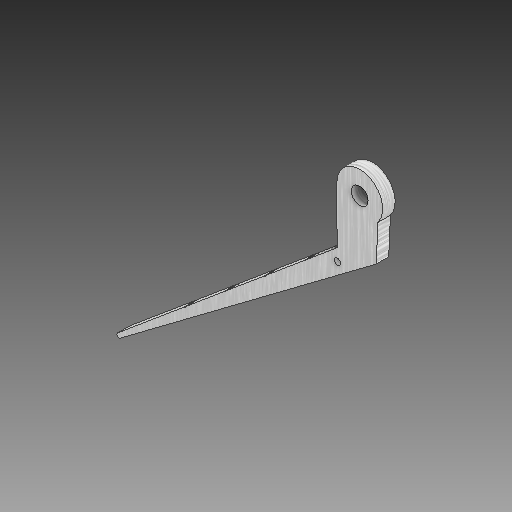
# Autodesk Inventor part: アームシールド根本1
Saved by Autodesk Inventor 2020 (Build 240168000, 168)
## iProperties
Created: 2019-09-16
Part Number: アームシールド根本1
Material: アルミニウム 7075
Document SubType Name: Modeling
Designer: 雪村
Density: 2.81 g/cm^3
Appearance: サテン - ブラシ仕上げ 重厚
Mass: 24.6363 g
Surface Area: 56.0611 cm^2
Volume: 8.76735 cm^3
Author: 雪村
Autodesk Inventor part; units mm, degrees
ref_plane "YZ Plane" through (0, 0, 0) normal (1, 0, 0) x (0, 1, 0)
ref_plane "XZ Plane" through (0, 0, 0) normal (0, 1, 0) x (-1, 0, 0)
ref_plane "XY Plane" through (0, 0, 0) normal (0, 0, 1) x (1, 0, 0)
sketch "スケッチ1" plane through (0, 0, 0) normal (0, 0, 1) x (1, 0, 0)
  circle A0 centre (-149.101, -13.3308) radius 1.5 construction
  circle A1 centre (-160.5892, -1.6149) radius 1.5 construction
  circle A2 centre (-44.4492, 64.0137) radius 1.5 construction
  circle A3 centre (-64.4423, 49.0046) radius 1.5 construction
  circle A4 centre (-60.4494, 64.5064) radius 1.5 construction
  arc A5 (-40.2316, 58.3956) -> (-44.233, 71.0354) centre (-44.4492, 64.0137) ccw construction
  line L0 (-44.233, 71.0354) -> (-60.2332, 71.5281) construction
  arc A6 (-60.2332, 71.5281) -> (-64.1725, 70.4637) centre (-60.4494, 64.5064) ccw construction
  line L1 (-64.1725, 70.4637) -> (-165.9022, 6.8864) construction
  arc A7 (-165.9022, 6.8864) -> (-166.8262, -9.4635) centre (-160.5892, -1.6149) ccw construction
  line L2 (-166.8262, -9.4635) -> (-154.0782, -19.594) construction
  arc A8 (-154.0782, -19.594) -> (-144.2981, -19.7286) centre (-149.101, -13.3308) ccw construction
  line L3 (-144.2981, -19.7286) -> (-40.2316, 58.3956) construction
  circle A9 centre (-82.1645, 51.5544) radius 1.5 construction
  circle A10 centre (-141.748, 14.817) radius 1.5 construction
  circle A11 centre (-89.4637, 29.5642) radius 1.5 construction
  circle A12 centre (-117.4541, 8.5514) radius 1.5 construction
  circle A13 centre (-111.8449, 33.0052) radius 1.5 construction
  line L4 (-152.7009, -26.0367) -> (-305.9655, -141.0946)
  circle A14 centre (-149.101, -13.3308) radius 1.5 construction
  circle A15 centre (-149.101, -13.3308) radius 3 construction
  circle A16 centre (-149.101, -13.3308) radius 3 construction
  circle A17 centre (-160.5892, -1.6149) radius 9.025 construction
  circle A18 centre (-160.5892, -1.6149) radius 4.025
  line L5 (-152.7009, -26.0367) -> (-151.5741, -2.0382)
  line L6 (-64.1725, 70.4637) -> (-165.9022, 6.8864) construction
  line L7 (-144.2981, -19.7286) -> (-40.2316, 58.3956) construction
  line L8 (-305.9655, -141.0946) -> (-171.4423, -28.6314)
  line L9 (-160.5892, -1.6149) -> (-146.0204, -21.0215) construction
  line L10 (-146.0204, -21.0215) -> (-305.9655, -141.0946) construction
  circle A19 centre (-276.0256, -117.3678) radius 1
  circle A20 centre (-160.5892, -1.6149) radius 11
  line L11 (-171.4423, -28.6314) -> (-171.589, -1.6748)
  point P0 (0, 0)
  point P1 (0, 0)
  point P2 (-276.667, -116.6006)
  point P3 (-275.4252, -118.1676)
  point P4 (-151.8691, -8.3201)
  dimension "d6" = 22
  dimension "d0" = 6
  dimension "d1" = 8.05
  dimension "d2" = 5
  dimension "d3" = 3
  dimension "d4" = 200
  dimension "d5" = 2
  dimension "d7" = 3
  dimension "d8" = 6
  constraints: 24 end point, 19 centre point, 8 point on circle, 4 tangent, 3 coincident, 2 collinear, 2 concentric, 1 perpendicular, 42 other
  measures "d0" diameter of A15
  measures "d1" diameter of A18
  measures "d3" angle of L4 L8
  measures "d4" distance of L9.end L4.end
  measures "d5" diameter of A19
  measures "d7" angle of L5 L11
  measures "d8" diameter of A16
extrude "押し出し1" add sketch "スケッチ1" along normal blind 6 contours L4 A19 L8 L11 A20 L5 | A19 | A20
sketch "スケッチ2" plane through (0, 0, 6) normal (0, 0, 1) x (1, 0, 0)
  line L0 (-171.589, -1.6748) -> (-171.4423, -28.6314) projected
  line L1 (-171.4423, -28.6314) -> (-276.667, -116.6006) projected
  arc A0 (-276.667, -116.6006) -> (-275.4252, -118.1676) centre (-276.0256, -117.3678) ccw projected
  line L2 (-275.4252, -118.1676) -> (-152.7009, -26.0367) projected
  line L3 (-152.7009, -26.0367) -> (-151.8691, -8.3201) projected
  arc A1 (-151.8691, -8.3201) -> (-171.589, -1.6748) centre (-160.5892, -1.6149) ccw projected
  circle A2 centre (-160.5892, -1.6149) radius 4.025 projected
  circle A3 centre (-171.2358, -34.3242) radius 1.5
  circle A4 centre (-171.2358, -34.3242) radius 3
  circle A5 centre (-171.2358, -34.3242) radius 4.5
  point P0 (0, 0)
  dimension "d11" = 3
  dimension "d12" = 6
  dimension "d13" = 9
  constraints: 3 centre point, 2 coincident, 2 tangent
  measures "d11" diameter of A3
  measures "d12" diameter of A4
  measures "d13" diameter of A5
extrude "押し出し2" cut sketch "スケッチ2" against normal through all contours A3
sketch "スケッチ3" plane through (0, 0, 6) normal (0, 0, 1) x (1, 0, 0)
  line L0 (-171.4423, -28.6314) -> (-276.667, -116.6006) projected
  circle A0 centre (-244.7975, -88.9797) radius 1.05
  circle A1 centre (-225.6172, -72.9448) radius 1.05
  circle A2 centre (-206.437, -56.9099) radius 1.05
  circle A3 centre (-187.2568, -40.8749) radius 1.05
  point P0 (0, 0)
  dimension "d16" = 2.1
  dimension "d17" = 2.1
  dimension "d18" = 2.1
  dimension "d19" = 2.1
  dimension "d20" = 0.75
  dimension "d21" = 0.75
  dimension "d22" = 0.75
  dimension "d23" = 0.75
  dimension "d24" = 20
  dimension "d25" = 25
  dimension "d26" = 25
  dimension "d27" = 25
  constraints: 4 centre point
  measures "d16" diameter of A0
  measures "d17" diameter of A1
  measures "d18" diameter of A2
  measures "d19" diameter of A3
  measures "d20" distance from line of L0 A3.centre
  measures "d21" distance from line of L0 A2.centre
  measures "d22" distance from line of L0 A0.centre
  measures "d23" distance from line of L0 A1.centre
  measures "d24" distance of A3.centre L0.start
  measures "d25" distance of A2.centre A3.centre
  measures "d26" distance of A1.centre A2.centre
  measures "d27" distance of A1.centre A0.centre
extrude "押し出し3" cut sketch "スケッチ3" against normal through all
sketch "スケッチ4" plane through (-205.3922, -57.0139, 6) normal (-0.6413971, 0.7672091, 0) x (0.7672091, 0.6413971, 0)
  line L0 (-25, 6) -> (-25, 0) projected
  line L1 (-1.4697, 0) -> (-25, 0) projected
  line L2 (-1.4697, 0) -> (-1.4697, 6) projected
  line L3 (-1.4697, 6) -> (-25, 6) projected
  line L4 (-26.4697, 0) -> (-26.4697, 6) projected
  line L5 (-26.4697, 6) -> (-50, 6) projected
  line L6 (-50, 6) -> (-50, 0) projected
  line L7 (-26.4697, 0) -> (-50, 0) projected
  line L8 (-51.4697, 0) -> (-51.4697, 6) projected
  line L9 (-51.4697, 6) -> (-92.9014, 6) projected
  line L10 (-92.9014, 6) -> (-92.9014, 0) projected
  line L11 (-51.4697, 0) -> (-92.9014, 0) projected
  line L12 (0, 6) -> (0, 0) projected
  line L13 (23.5303, 0) -> (0, 0) projected
  line L14 (23.5303, 0) -> (23.5303, 6) projected
  line L15 (23.5303, 6) -> (0, 6) projected
  line L16 (25, 6) -> (25, 0) projected
  line L17 (44.2511, 0) -> (25, 0) projected
  line L18 (44.2511, 6) -> (44.2511, 0) projected
  line L19 (44.2511, 6) -> (25, 6) projected
  circle A0 centre (-50.7348, 3) radius 1.25
  circle A1 centre (-25.7348, 3) radius 1.25
  circle A2 centre (-0.7348, 3) radius 1.25
  circle A3 centre (24.2652, 3) radius 1.25
  line L20 (23.5303, 6) -> (25, 6) projected
  line L21 (-1.4697, 6) -> (0, 6) projected
  line L22 (-26.4697, 6) -> (-25, 6) projected
  line L23 (-51.4697, 6) -> (-50, 6) projected
  point P0 (194.1473, 6)
  point P1 (-51.4697, 3)
  point P2 (-26.4697, 3)
  point P3 (-50.7348, 6)
  point P4 (-25.7348, 6)
  point P5 (-0.7348, 6)
  point P6 (24.2652, 6)
  point P7 (23.5303, 3)
  point P8 (-1.4697, 3)
  dimension "d30" = 2.5
  dimension "d31" = 2.5
  dimension "d32" = 2.5
  dimension "d33" = 2.5
  constraints: 8 midpoint, 4 centre point, 4 horizontal alignment, 4 vertical alignment
  measures "d30" diameter of A0
  measures "d31" diameter of A1
  measures "d32" diameter of A2
  measures "d33" diameter of A3
extrude "押し出し4" cut sketch "スケッチ4" against normal through all contours A1 L0 | L0 A1 L4 | L4 A1 | A2 L12 L2 | L2 A2 | A2 L12 | A0 L6 | L6 A0 L8 | A3 L16 L14 | L14 A3 | L8 A0 | A3 L16
sketch "スケッチ5" plane through (0, 0, 6) normal (0, 0, 1) x (1, 0, 0)
  arc A0 (-225.7, -73.9915) -> (-224.5724, -73.0489) centre (-225.6172, -72.9448) ccw projected
  line L0 (-225.7, -73.9915) -> (-243.7526, -89.0838) projected
  arc A1 (-244.8802, -90.0264) -> (-243.7526, -89.0838) centre (-244.7975, -88.9797) ccw projected
  line L1 (-244.8802, -90.0264) -> (-276.667, -116.6006) projected
  arc A2 (-276.667, -116.6006) -> (-275.4252, -118.1676) centre (-276.0256, -117.3678) ccw projected
  line L2 (-275.4252, -118.1676) -> (-152.7009, -26.0367) projected
  line L3 (-152.7009, -26.0367) -> (-151.8691, -8.3201) projected
  arc A3 (-151.8691, -8.3201) -> (-171.589, -1.6748) centre (-160.5892, -1.6149) ccw projected
  line L4 (-171.589, -1.6748) -> (-171.4423, -28.6314) projected
  line L5 (-171.4423, -28.6314) -> (-186.2119, -40.979) projected
  arc A4 (-187.3395, -41.9217) -> (-186.2119, -40.979) centre (-187.2568, -40.8749) ccw projected
  line L6 (-187.3395, -41.9217) -> (-205.3922, -57.0139) projected
  arc A5 (-206.5197, -57.9566) -> (-205.3922, -57.0139) centre (-206.437, -56.9099) ccw projected
  line L7 (-206.5197, -57.9566) -> (-224.5724, -73.0489) projected
  circle A6 centre (-171.2358, -34.3242) radius 1.5 projected
  circle A7 centre (-160.5892, -1.6149) radius 4.025 projected
  point P0 (0, 0)
equation "\"d8\" = d0"
equation "\"d21\" = d20"
equation "\"d22\" = d21"
equation "\"d23\" = d21"
equation "\"d26\" = d25"
equation "\"d27\" = d26"
